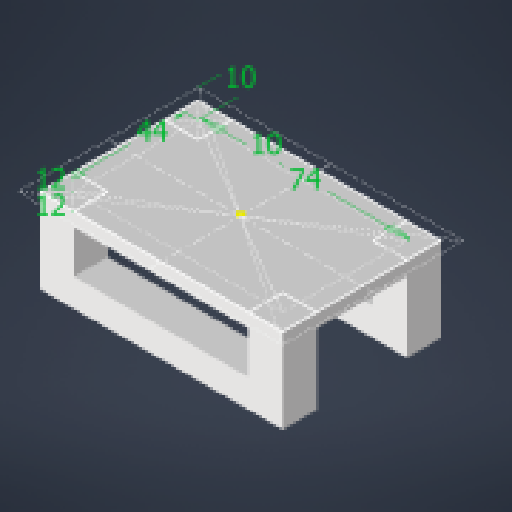
# Autodesk Inventor part: PCB_Housing_01
Saved by Autodesk Inventor 2026.2 (Build 302298000, 298)
## iProperties
Created: 2026-02-04
Part Number: PCB_Housing_01
Material: Generic
Document SubType Name: Modeling
Designer: vckot
Density: 1 g/cm^3
Appearance: Default
Author: vckot
Autodesk Inventor part; units mm, degrees
ref_plane "YZ Plane" through (0, 0, 0) normal (1, 0, 0) x (0, 1, 0)
ref_plane "XZ Plane" through (0, 0, 0) normal (0, 1, 0) x (-1, 0, 0)
ref_plane "XY Plane" through (0, 0, 0) normal (0, 0, 1) x (1, 0, 0)
sketch "Sketch1" plane through (0, 0, 0) normal (0, 1, 0) x (-1, 0, 0)
  line L0 (-37, 22) -> (37, 22) construction
  line L1 (37, 22) -> (37, -22) construction
  line L2 (37, -22) -> (-37, -22) construction
  line L3 (-37, -22) -> (-37, 22) construction
  line L4 (-37, 22) -> (37, -22) construction
  line L5 (37, 22) -> (-37, -22) construction
  line L6 (-47, 32) -> (47, 32) construction
  line L7 (47, 32) -> (47, -32) construction
  line L8 (47, -32) -> (-47, -32) construction
  line L9 (-47, -32) -> (-47, 32) construction
  line L10 (-47, 32) -> (47, -32) construction
  line L11 (47, 32) -> (-47, -32) construction
  line L12 (31, 16) -> (43, 16)
  line L13 (43, 16) -> (43, 28)
  line L14 (43, 28) -> (31, 28)
  line L15 (31, 28) -> (31, 16)
  line L16 (31, 16) -> (43, 28) construction
  line L17 (43, 16) -> (31, 28) construction
  line L18 (47, 0) -> (-47, 0) construction
  line L19 (0, 32) -> (0, -32) construction
  line L20 (37, -22) -> (-37, 22) construction
  line L21 (47, -32) -> (-47, 32) construction
  line L22 (31, -16) -> (43, -16)
  line L23 (43, -16) -> (43, -28)
  line L24 (43, -28) -> (31, -28)
  line L25 (31, -28) -> (31, -16)
  line L26 (31, -16) -> (43, -28) construction
  line L27 (43, -16) -> (31, -28) construction
  line L28 (-31, 16) -> (-43, 16)
  line L29 (-43, 16) -> (-43, 28)
  line L30 (-43, 28) -> (-31, 28)
  line L31 (-31, 28) -> (-31, 16)
  line L32 (-31, -16) -> (-43, -16)
  line L33 (-31, -28) -> (-31, -16)
  line L34 (-43, -28) -> (-31, -28)
  line L35 (-43, -16) -> (-43, -28)
  line L36 (43, 28) -> (-43, 28)
  line L37 (-43, 28) -> (-43, -28)
  line L38 (-43, -28) -> (43, -28)
  line L39 (43, -28) -> (43, 28)
  point P0 (0, 0)
  dimension "d0" = 74
  dimension "d1" = 44
  dimension "d2" = 10
  dimension "d3" = 10
  dimension "d4" = 12
  dimension "d5" = 12
  constraints: 80 end point, 12 symmetric about line, 10 midpoint, 8 parallel, 4 horizontal, 4 perpendicular
  measures "d0" distance of L1.end L2.end
  measures "d1" distance of L0.end L1.end
  measures "d2" distance between parallel lines of L8 L2
  measures "d3" distance between parallel lines of L7 L1
  measures "d4" distance of L14.end L13.end
  measures "d5" distance of L13.end L12.end
extrude "Extrusion1" add sketch "Sketch1" against normal blind 5
extrude "Extrusion2" add sketch "Sketch1" against normal blind 30 contours L15 L14 L13 L12 | L23 L24 L25 L22 | L31 L28 L29 L30 | L34 L35 L32 L33
hole "Hole2" at (-37, 0, 22) at (-37, 0, -22) at (37, 0, -22) at (37, 0, 22) direction (0, -1, 0) diameter 2.4 depth 8 tip angle 118 clearance for "Flat Head Machine Screw" size "M2" standard "Ansi Metric M Profile"
sketch "Sketch4" plane through (0, -30, 0) normal (0, -1, 0) x (1, 0, 0)
  line L0 (31, 28) -> (-31, 28) projected
  line L1 (-43, 16) -> (-31, 16) projected
  line L2 (31, 28) -> (-31, 28)
  line L3 (-31, 28) -> (-31, 16)
  line L4 (-31, 16) -> (31, 16)
  line L5 (31, 16) -> (31, 28)
  line L6 (43, -28) -> (-43, -28) projected
  line L7 (-43, -16) -> (-31, -16) projected
  line L8 (31, -28) -> (-31, -28)
  line L9 (-31, -28) -> (-31, -16)
  line L10 (-31, -16) -> (31, -16)
  line L11 (31, -16) -> (31, -28)
  point P0 (0, 0)
  constraints: 16 end point, 4 parallel, 2 horizontal, 2 perpendicular, 2 point on line
extrude "Extrusion3" add sketch "Sketch4" against normal blind 10
body "Solid1"
